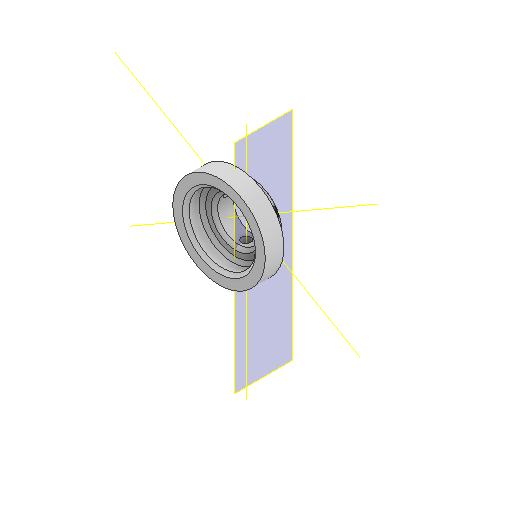
# Autodesk Inventor part: 30_Linear_Stage_NEMA11_baseholder_bayonetmount_objective_v0
Saved by Autodesk Inventor 2022 (Build 260153000, 153)
## iProperties
Created: 2023-02-17
Part Number: 30_Linear_Stage_NEMA11_baseholder_bayonetmount_objective_v0
Material: Generisch
Document SubType Name: Modeling
Designer: diederichbenedict
Density: 1 g/cm^3
Appearance: Vorgabe
Vendor: openUC2
Author: diederichbenedict
Autodesk Inventor part; units mm, degrees
ref_plane "YZ Plane" through (0, 0, 0) normal (1, 0, 0) x (0, 1, 0)
ref_plane "XZ Plane" through (0, 0, 0) normal (0, 1, 0) x (-1, 0, 0)
ref_plane "XY Plane" through (0, 0, 0) normal (0, 0, 1) x (1, 0, 0)
ref_plane "Arbeitsebene1" through (15, 0, 0) normal (-1, 0, 0) x (0, 1, 0)
sketch "Skizze1" plane through (15, 0, 0) normal (-1, 0, 0) x (0, 1, 0)
  line L0 (32.6031, 0.5) -> (30.7237, 0.5) projected
  line L1 (30.7237, 4.25) -> (32.6031, 4.25) projected
  line L2 (30.7237, 0.5) -> (30.7237, 4.25) projected
  line L3 (32.6031, 0.5) -> (30.7237, 0.5) projected
  line L4 (30.7237, 4.7) -> (32.6031, 4.7) projected
  line L5 (30.7237, 0.5) -> (30.7237, 4.25) projected
  line L6 (30, 0.5) -> (32, 0.5) projected
  line L7 (30, 0.55) -> (30, 0.5) projected
  line L8 (32, 0.5) -> (32, 0.55) projected
  line L9 (32, 0.5) -> (32, 16.1)
  line L10 (52, 0.5) -> (52, 16.1)
  line L11 (42, 19.32) -> (42, -3.22)
  line L12 (32.6031, 0.5) -> (28, 0.5)
  line L13 (28, 0.5) -> (28, -5.5)
  line L14 (28, -5.5) -> (35.6031, -5.5)
  line L15 (35.6031, -5.5) -> (35.6031, 5.25)
  line L16 (35.6031, 5.25) -> (34.1031, 5.25)
  line L17 (32.6031, 0.5) -> (32.6031, 0.2)
  line L18 (32.6031, 0.2) -> (28, 0.2)
  line L19 (32, 0.55) -> (30, 0.55) projected
  line L20 (32.1031, 0.5) -> (32.0412, 0.2)
  line L21 (28, -5.5) -> (32, -5.5)
  line L22 (32, -5.5) -> (32, -13.5)
  line L23 (32, -13.5) -> (28, -13.5)
  line L24 (28, -13.5) -> (28, -5.5)
  line L25 (34.1031, 5.25) -> (32.307, 3.9176)
  line L26 (32.307, 3.9176) -> (32.1031, 0.5)
  point P0 (0, 0)
  dimension "d1" = 6
  dimension "d3" = 1
  dimension "d11" = 0.5
  dimension "d13" = 14
  dimension "d14" = 8
  dimension "d15" = 10
  dimension "d37" = 0.3
  dimension "d38" = 6.3969
  constraints: 34 end point, 5 perpendicular, 4 vertical, 3 point on line, 2 parallel, 1 coincident, 1 collinear, 1 horizontal, 5 other
  measures "d1" distance between parallel lines of L12 L14
  measures "d3" distance between parallel lines of L1 L16
  measures "d11" distance of L0.start L20.start
  measures "d13" distance between parallel lines of L13 L11
  measures "d14" distance of L21.end L22.end
  measures "d15" distance between parallel lines of L11 L22
  measures "d37" distance between parallel lines of L18 L0
  measures "d38" distance between parallel lines of L15 L11
revolve "Umdrehung1" add sketch "Skizze1" angle 360 about axis through (15, 42, -19.32) along (0, 0, 1) contours L17 L18 L20 L0 | L0 L26 L25 L16 L15 L14 L13 L18 L17
sketch "Skizze2" plane through (0, 0, 0) normal (0, 1, 0) x (-1, 0, 0)
  spline S0 degree 3 poles (-15, -4.25) (-12.1304, -4.4784) (-9.2732, -4.7067) (-7.1109, -4.9351) (-6.8554, -4.962) (-6.6095, -4.989) (-6.3738, -5.016) knots 0 0 0 0 0.7174 0.7174 0.7174 0.802142 0.802142 0.802142 0.802142 projected
  spline S1 degree 3 poles (-14.5016, -1.0897) (-11.6314, -1.3183) (-8.8183, -1.5469) (-6.7355, -1.7755) (-6.2054, -1.8336) (-5.7215, -1.8918) (-5.2918, -1.95) knots 0.041547 0.041547 0.041547 0.041547 0.759706 0.759706 0.759706 0.942478 0.942478 0.942478 0.942478 projected
  circle A0 centre (-15, -2.8138) radius 1.4
  line L0 (-15, 1.0048) -> (-15, -6.0288) projected
  point P0 (0, 0)
  dimension "d5" = 2.8
  constraints: 1 centre point, 1 point on line
  measures "d5" diameter of A0
extrude "Extrusion1" cut sketch "Skizze2" along normal up to surface
pattern_circular "Runde Anordnung1" count 3 over 360 about axis through (15, 42, 2.65) along (0, 0, -1) of "Extrusion1"
chamfer "Fase1" distance 1 angle 45 1 edges at (15, 48.3969, 5.5)
sketch "Skizze6" plane through (15, 42, 5.5) normal (0, 0, 1) x (1, 0, 0)
  circle A0 centre (0, 0) radius 14 projected
  circle A1 centre (0, 0) radius 7.3969 projected
  circle A2 centre (0, 0) radius 10.05
  point P0 (-15, -42)
  dimension "d31" = 20.1
  constraints: 1 centre point, 1 coincident
  measures "d31" diameter of A2
extrude "Extrusion4" cut sketch "Skizze6" against normal blind 5 contours A1 | A2
chamfer "Fase3" distance 1 angle 45 3 edges at (15, 48.3969, 0.5) (4.95, 42, 5.5) (4.95, 42, 0.5)
